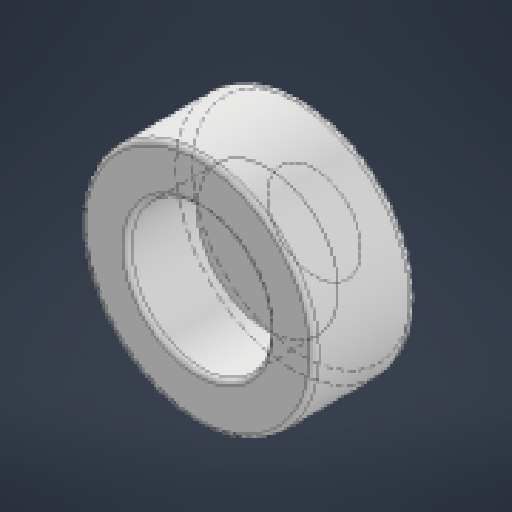
# Autodesk Inventor part: FOOT
Saved by Autodesk Inventor 2023 (Build 270158000, 158)
## iProperties
Created: 2025-09-04
Part Number: FOOT
Material: 일반
Document SubType Name: Modeling
Designer: k
Density: 1 g/cm^3
Appearance: 기본값
Author: k
Autodesk Inventor part; units mm, degrees
ref_plane "YZ Plane" through (0, 0, 0) normal (1, 0, 0) x (0, 1, 0)
ref_plane "XZ Plane" through (0, 0, 0) normal (0, 1, 0) x (-1, 0, 0)
ref_plane "XY Plane" through (0, 0, 0) normal (0, 0, 1) x (1, 0, 0)
sketch "스케치1" plane through (0, 0, 0) normal (1, 0, 0) x (0, 1, 0)
  line L0 (50.1069, 54.6508) -> (50.1069, -12.84)
  line L1 (75.1069, 20.7597) -> (75.1069, 1.3993)
  line L2 (59.8099, -3.2403) -> (40.1069, -3.2403)
  line L3 (25.1069, 1.3993) -> (25.1069, 20.7597)
  line L4 (35.0069, 6.7597) -> (65.2069, 6.7597)
  line L5 (26.7147, -0.5618) -> (40.1069, -3.2403)
  line L6 (73.4992, -0.5618) -> (60.3982, -3.182)
  line L7 (26.1069, 21.7597) -> (34.0069, 21.7597)
  line L8 (66.2069, 21.7597) -> (74.1069, 21.7597)
  line L9 (35.0069, 20.7597) -> (35.0069, 6.7597)
  line L10 (65.2069, 20.7597) -> (65.2069, 6.7597)
  arc A0 (25.1069, 1.3993) -> (26.7147, -0.5618) centre (27.1069, 1.3993) ccw
  arc A1 (73.4992, -0.5618) -> (75.1069, 1.3993) centre (73.1069, 1.3993) ccw
  arc A2 (25.1069, 1.3993) -> (26.7147, -0.5618) centre (27.1069, 1.3993) ccw
  arc A3 (26.1069, 21.7597) -> (25.1069, 20.7597) centre (26.1069, 20.7597) ccw
  arc A4 (35.0069, 20.7597) -> (34.0069, 21.7597) centre (34.0069, 20.7597) ccw
  arc A5 (66.2069, 21.7597) -> (65.2069, 20.7597) centre (66.2069, 20.7597) ccw
  arc A6 (75.1069, 20.7597) -> (74.1069, 21.7597) centre (74.1069, 20.7597) ccw
  point P0 (0, 0)
  point P1 (25.1069, 21.7597)
  point P2 (75.1069, 21.7597)
  point P3 (50.1069, -3.2403)
  point P4 (50.1069, 6.7597)
  dimension "d0" = 50
  dimension "d2" = 25
  dimension "d6" = 30.2
  dimension "d7" = 15.1
  dimension "d8" = 25
  dimension "d10" = 2
  dimension "d11" = 2
  dimension "d12" = 1
  dimension "d13" = 1
  dimension "d14" = 1
  constraints: 22 end point, 14 point on circle, 14 tangent, 7 centre point, 6 point on line, 5 parallel, 3 horizontal, 2 equal radius, 2 perpendicular, 1 vertical
  measures "d0" distance of point (25.107, 21.76) point (75.107, 21.76)
  measures "d2" distance between parallel lines of L0 L3
  measures "d6" distance between parallel lines of L10 L9
  measures "d7" distance between parallel lines of L0 L10
  measures "d8" distance between parallel lines of L8 L2
  measures "d10" radius of A0
  measures "d11" radius of A1
  measures "d12" radius of A3
  measures "d13" radius of A5
  measures "d14" radius of A6
revolve "회전1" add sketch "스케치1" angle 360 about axis through (0, 50.1069, 54.6508) along (0, 0, -1)
